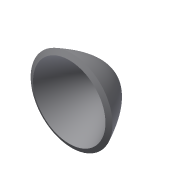
# Autodesk Inventor part: bowl
Saved by Autodesk Inventor 2015 (Build 190159000, 159)
## iProperties
Created: 2014-10-03
Part Number: bowl
Material: Generic
Document SubType Name: Modeling
Designer: Peter
Density: 1 g/cm^3
Appearance: Default
Author: Peter
Autodesk Inventor part; units mm, degrees
ref_plane "YZ Plane" through (0, 0, 0) normal (1, 0, 0) x (0, 1, 0)
ref_plane "XZ Plane" through (0, 0, 0) normal (0, 1, 0) x (-1, 0, 0)
ref_plane "XY Plane" through (0, 0, 0) normal (0, 0, 1) x (1, 0, 0)
sketch "Sketch2" plane through (0, 0, 0) normal (1, 0, 0) x (0, 1, 0)
  spline S0 degree 5 poles (0, 0) (7.9252, 0.0002) (15.8579, 1.0297) (23.5911, 3.0959) (39.9646, 9.4606) (54.7305, 19.0433) (62.2954, 24.9474) (78.5555, 39.4958) (92.865, 55.9897) (100.3984, 65.625) (116.485, 88.056) (130.7996, 111.6655) (138.3443, 125.063) (145.527, 138.6542) (152.4, 152.4) knots 0 0 0 0 0 0 0.17584 0.17584 0.17584 0.388045 0.388045 0.388045 0.659073 0.659073 0.659073 1 1 1 1 1 1
  line L0 (0, 0) -> (0, -22.225)
  line L1 (152.4, 152.4) -> (172.2786, 142.4607)
  spline S1 degree 5 poles (0.0006, -22.225) (9.486, -22.2244) (18.9759, -21.0841) (28.2702, -18.7919) (45.4799, -12.514) (61.2688, -3.244) (68.4843, 1.7564) (81.8275, 12.3068) (93.9952, 24.1892) (99.6399, 30.1928) (110.3012, 42.399) (120.175, 55.2497) (124.8603, 61.6956) (133.8431, 74.6837) (142.2809, 88.0323) (146.3409, 94.7207) (154.1994, 108.1546) (161.6596, 121.8137) (165.2799, 128.6547) (168.8175, 135.5385) (172.2786, 142.4606) knots 0 0 0 0 0 0 0.189726 0.189726 0.189726 0.364788 0.364788 0.364788 0.529442 0.529442 0.529442 0.688757 0.688757 0.688757 0.845215 0.845215 0.845215 1 1 1 1 1 1
  dimension "d4" = 22.225
  dimension "d5" = 63.435
  constraints: 4 end point, 1 vertical, 8 other
  measures "d5" angle of L0 L1
revolve "Revolution1" add sketch "Sketch2" angle 360 about axis through (0, 0, 0) along (0, 0, -1)
equation "curve S0 of \"Sketch2\": x = t; y = t^2/6; t from d2 to d3"
body "Solid1"
